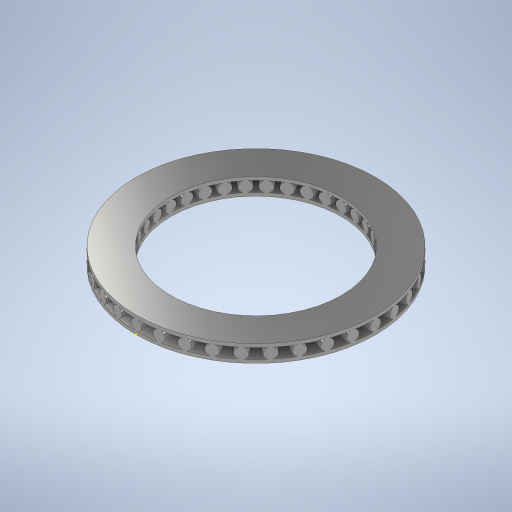
# Autodesk Inventor part: AXK5070+AS Bearing
Saved by Autodesk Inventor 2024.1 (Build 281209000, 209)
## iProperties
Created: 2023-09-08
Part Number: AXK5070+AS Bearing
Material: Stainless Steel
Document SubType Name: Modeling
Designer: chanh
Density: 8 g/cm^3
Appearance: Semi-Polished
Author: chanh
Autodesk Inventor part; units mm, degrees
ref_plane "YZ Plane" through (0, 0, 0) normal (1, 0, 0) x (0, 1, 0)
sketch "Sketch1" plane through (0, 0, 0) normal (0, 1, 0) x (-1, 0, 0)
  circle A0 centre (0, 0) radius 35
  circle A1 centre (0, 0) radius 25
  dimension "d0" = 70
  dimension "d1" = 50
  constraints: 2 centre point, 2 coincident
  measures "d0" diameter of A0
  measures "d1" diameter of A1
extrude "Extrusion1" add sketch "Sketch1" along normal blind 1
ref_plane "Work Plane1" through (0, 0, 35) normal (0, 0, 1) x (1, 0, 0)
sketch "Sketch2" plane through (0, 0, 35) normal (0, 0, 1) x (1, 0, 0)
  line L0 (35, 1) -> (-35, 1) projected
  circle A0 centre (0, 2.5) radius 1.6
  point P0 (0, 0)
  point P1 (0.5568, 1)
  point P2 (-0.5568, 1)
  dimension "d4" = 3.2
  dimension "d5" = 2.5
  constraints: 1 centre point, 1 vertical alignment
  measures "d4" diameter of A0
  measures "d5" distance of A0.centre point (0, 0)
extrude "Extrusion2" add sketch "Sketch2" against normal blind 11.5875 contours L0 A0 picked at (0.6109, 1.9988)
pattern_circular "Circular Pattern1" count 36 over 360 about axis through (0, -10, 0) along (0, 1, 0) of "Extrusion2"
sketch "Sketch3" plane through (0, 0, 35) normal (0, 0, 1) x (1, 0, 0)
  point P0 (0, 0)
ref_plane "Work Plane3" through (0, 4, 35) normal (0, 1, 0) x (1, 0, 0)
ref_plane "Work Plane2" through (0, 4.1, 35) normal (0, 1, 0) x (1, 0, 0)
sketch "Sketch4" plane through (0, 4, 35) normal (0, 1, 0) x (1, 0, 0)
  circle A0 centre (0, 35) radius 25 projected
  circle A1 centre (0, 35) radius 35 projected
extrude "Extrusion3" add sketch "Sketch4" along normal blind 1
sketch "Sketch5" plane through (0, 5, 0) normal (0, 1, 0) x (1, 0, 0)
  circle A0 centre (0, 0) radius 25 projected
  circle A1 centre (0, 0) radius 35 projected
  circle A2 centre (0, 0) radius 40
  dimension "d14" = 5
  constraints: 1 centre point
  measures "d14" radial gap between concentric circles of A1 A2
extrude "Extrusion4" cut sketch "Sketch5" against normal through all
body "Solid1"
